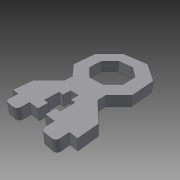
# Autodesk Inventor part: filament_guide
Saved by Autodesk Inventor 2014 (Build 180170000, 170)
## iProperties
Created: 2013-12-07
Part Number: filament_guide
Material: Generic
Document SubType Name: Modeling
Designer: buben
Density: 1 g/cm^3
Appearance: Default
Author: buben
Subject: Laser Cutted
Autodesk Inventor part; units mm, degrees
ref_plane "YZ Plane" through (0, 0, 0) normal (1, 0, 0) x (0, 1, 0)
ref_plane "XZ Plane" through (0, 0, 0) normal (0, 1, 0) x (-1, 0, 0)
ref_plane "XY Plane" through (0, 0, 0) normal (0, 0, 1) x (1, 0, 0)
sketch "Sketch1" plane through (0, 0, 0) normal (0, 0, 1) x (1, 0, 0)
  line L0 (0, 0) -> (39, 0)
  line L1 (0, 0) -> (0, 10)
  line L2 (39, 0) -> (39, 10)
  line L3 (0, 10) -> (9.5, 19.5)
  line L4 (39, 10) -> (29.5, 19.5)
  line L5 (9.5, 24.2513) -> (2, 31.7513)
  line L6 (2, 31.7513) -> (2, 46.2487)
  line L7 (2, 46.2487) -> (12.2513, 56.5)
  line L8 (12.2513, 56.5) -> (26.7487, 56.5)
  line L9 (26.7487, 56.5) -> (37, 46.2487)
  line L10 (37, 46.2487) -> (37, 31.7513)
  line L11 (37, 31.7513) -> (29.5, 24.2513)
  line L12 (23.6421, 29) -> (15.3579, 29)
  line L13 (15.3579, 29) -> (9.5, 34.8579)
  line L14 (9.5, 34.8579) -> (9.5, 43.1421)
  line L15 (9.5, 43.1421) -> (15.3579, 49)
  line L16 (15.3579, 49) -> (23.6421, 49)
  line L17 (23.6421, 49) -> (29.5, 43.1421)
  line L18 (29.5, 43.1421) -> (29.5, 34.8579)
  line L19 (29.5, 34.8579) -> (23.6421, 29)
  line L20 (9.5, 19.5) -> (9.5, 24.2513)
  line L21 (29.5, 19.5) -> (29.5, 24.2513)
  point P0 (19.5, 39)
  point P1 (19.5, 39)
  point P2 (19.5, 0)
  dimension "d0" = 39
  dimension "d1" = 45
  dimension "d2" = 39
  dimension "d3" = 20
  dimension "d4" = 35
  dimension "d5" = 10
  dimension "d6" = 20
  constraints: 44 end point, 3 horizontal alignment, 3 parallel, 3 perpendicular, 1 coincident, 1 horizontal, 1 midpoint, 1 vertical alignment, 29 other
  measures "d0" distance of L0.start L0.end
  measures "d1" angle of L3 L1
  measures "d2" distance from line of L0 point (19.5, 39)
  measures "d3" distance between parallel lines of L18 L14
  measures "d4" distance between parallel lines of L10 L6
  measures "d5" distance of L0.start L1.end
  measures "d6" distance between parallel lines of L21 L20
extrude "Extrusion1" add sketch "Sketch1" along normal blind 6
sketch "Sketch2" plane through (0, 0, 6) normal (0, 0, 1) x (1, 0, 0)
  line L0 (0, 0) -> (39, 0) projected
  line L1 (17.25, 16.3) -> (21.75, 16.3)
  line L2 (21.75, 0) -> (17.25, 0)
  line L3 (24.25, 12.3) -> (24.25, 5)
  line L4 (14.75, 5) -> (14.75, 12.3)
  line L5 (21.75, 16.3) -> (21.75, 12.3)
  line L6 (21.75, 5) -> (21.75, 0)
  line L7 (17.25, 0) -> (17.25, 5)
  line L8 (17.25, 12.3) -> (17.25, 16.3)
  line L9 (14.75, 12.3) -> (17.25, 12.3)
  line L10 (21.75, 12.3) -> (24.25, 12.3)
  line L11 (24.25, 5) -> (21.75, 5)
  line L12 (17.25, 5) -> (14.75, 5)
  point P0 (19.5, 16.3)
  point P1 (19.5, 0)
  dimension "d9" = 5
  dimension "d10" = 4
  dimension "d11" = 7.3
  dimension "d12" = 2.5
  dimension "d13" = 2.5
  dimension "d14" = 4.5
  constraints: 24 end point, 10 parallel, 5 collinear, 4 perpendicular, 3 horizontal, 2 midpoint, 1 vertical alignment
  measures "d9" distance of L2.end L7.end
  measures "d10" distance of L8.start L1.start
  measures "d11" distance of L4.start L4.end
  measures "d12" distance of L4.end L8.start
  measures "d13" distance of L5.end L3.start
  measures "d14" distance of L1.start L1.end
extrude "Extrusion2" cut sketch "Sketch2" against normal blind 6
sketch "Sketch3" plane through (0, 0, 6) normal (0, 0, 1) x (1, 0, 0)
  line L0 (21.75, 0) -> (39, 0) projected
  line L1 (0, 0) -> (17.25, 0) projected
  line L2 (17.25, 16.3) -> (21.75, 16.3) projected
  line L3 (4, 0) -> (12, 0)
  line L4 (12, 0) -> (12, -4)
  line L5 (10, -6) -> (6, -6)
  line L6 (4, -4) -> (4, 0)
  line L7 (27, 0) -> (35, 0)
  line L8 (35, 0) -> (35, -4)
  line L9 (33, -6) -> (29, -6)
  line L10 (27, -4) -> (27, 0)
  arc A0 (4, -4) -> (6, -6) centre (6, -4) ccw
  arc A1 (10, -6) -> (12, -4) centre (10, -4) ccw
  arc A2 (27, -4) -> (29, -6) centre (29, -4) ccw
  arc A3 (33, -6) -> (35, -4) centre (33, -4) ccw
  point P0 (19.5, 16.3)
  dimension "d17" = 2
  dimension "d18" = 8
  dimension "d19" = 8
  dimension "d20" = 6
  dimension "d21" = 7.5
  dimension "d22" = 15
  constraints: 16 end point, 8 point on circle, 8 tangent, 4 centre point, 4 parallel, 3 equal radius, 2 horizontal, 2 perpendicular, 2 point on line, 1 collinear, 1 midpoint
  measures "d17" radius of A0
  measures "d18" distance between parallel lines of L4 L6
  measures "d19" distance between parallel lines of L8 L10
  measures "d20" distance between parallel lines of L5 L3
  measures "d21" distance from line of point (19.5, 16.3) L4
  measures "d22" distance between parallel lines of L10 L4
extrude "Extrusion3" add sketch "Sketch3" against normal blind 6
body "Solid1"
